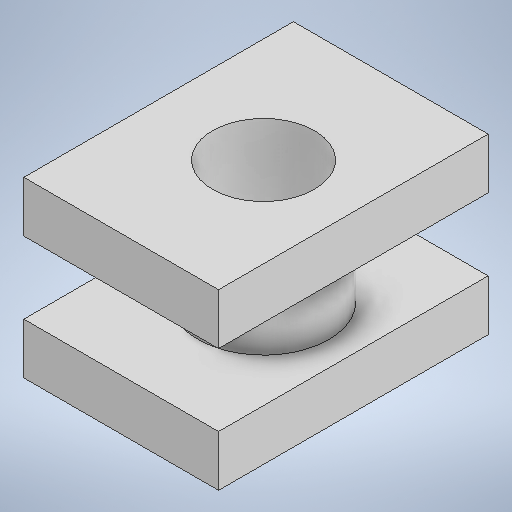
# Autodesk Inventor part: MMAE 232 Assignment 2_Rubber Grommet - Dylan Tamras
Saved by Autodesk Inventor 2025.2 (Build 292293000, 293)
## iProperties
Created: 2025-01-19
Part Number: MMAE 232 Assignment 2_Rubber Grommet - Dylan Tamras
Material: Generic
Document SubType Name: Modeling
Designer: Dylan
Density: 1 g/cm^3
Appearance: Default
Author: VRK99-0110
Title: Mechanical Component - 05
Autodesk Inventor part; units mm, degrees
ref_plane "YZ Plane" through (0, 0, 0) normal (1, 0, 0) x (0, 1, 0)
ref_plane "XZ Plane" through (0, 0, 0) normal (0, 1, 0) x (-1, 0, 0)
ref_plane "XY Plane" through (0, 0, 0) normal (0, 0, 1) x (1, 0, 0)
sketch "Sketch1" plane through (0, 0, 0) normal (0, 1, 0) x (-1, 0, 0)
  line L0 (0, 0) -> (6.5, 0)
  line L1 (6.5, 0) -> (6.5, -9)
  line L2 (6.5, -9) -> (0, -9)
  line L3 (0, 0) -> (0, -9)
  dimension "d0" = 6.5
  dimension "d1" = 9
  constraints: 8 end point, 2 perpendicular, 1 horizontal, 1 vertical
  measures "d0" distance of L0.start L0.end
  measures "d1" distance of L0.end L1.end
extrude "Extrusion1" add sketch "Sketch1" along normal blind 1.7
sketch "Sketch2" plane through (0, 1.7, 0) normal (0, 1, 0) x (1, 0, 0)
  circle A0 centre (-3, 4.5) radius 1.7
  dimension "d9" = 3.4
  constraints: 1 centre point
  measures "d9" diameter of A0
extrude "Extrusion2" cut sketch "Sketch2" against normal blind 1.7
sketch "Sketch3" plane through (0, 1.7, 0) normal (0, 1, 0) x (1, 0, 0)
  circle A0 centre (-3, 4.5) radius 2.18
  line L0 (-6.5, 3.2) -> (-4.75, 3.2)
  line L1 (-6.5, 5.8) -> (-4.75, 5.8)
  line L2 (-6.5, 3.2) -> (-6.5, 5.8)
  line L3 (-6.5, 9) -> (-6.5, 0) projected
  dimension "d12" = 4.36
  constraints: 6 end point, 2 point on circle, 1 centre point, 1 collinear, 1 horizontal, 1 parallel
  measures "d12" diameter of A0
extrude "Extrusion3" add sketch "Sketch3" along normal blind 2.4
sketch "Sketch4" plane through (0, 4.1, 0) normal (0, 1, 0) x (1, 0, 0)
  line L0 (-6.5, 0) -> (0, 0) projected
  line L1 (-6.5, 9) -> (-6.5, 5.8) projected
  line L2 (0, 0) -> (-6.5, 0)
  line L3 (-6.5, 0) -> (-6.5, 9)
  line L4 (-6.5, 9) -> (0, 9)
  line L5 (0, 9) -> (0, 0)
  constraints: 8 end point, 2 parallel, 1 horizontal, 1 perpendicular
extrude "Extrusion4" add sketch "Sketch4" along normal blind 1.7
sketch "Sketch5" plane through (0, 5.8, 0) normal (0, 1, 0) x (1, 0, 0)
  circle A0 centre (-3, 4.5) radius 1.7 projected
  circle A1 centre (-3, 4.5) radius 1.7
  dimension "d20" = 3.4
  constraints: 1 centre point, 1 coincident
  measures "d20" diameter of A1
extrude "Extrusion5" cut sketch "Sketch5" against normal blind 5.8
body "Solid1"
